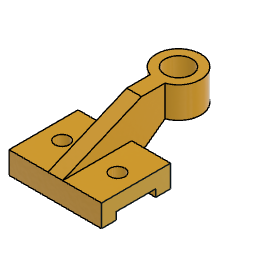
Part (Autodesk Fusion 360 design; units mm, degrees)
Autodesk Fusion 360 part; units mm, degrees
note: some values were not read from the file. Chosen so that the rebuilt part matches the saved one: a side.
sketch "Sketch1" plane through (0, 0, 0) normal (0, 1, 0) x (1, 0, 0)
  line L0 (0, 0) -> (31.5, 0)
  line L1 (31.5, 0) -> (31.5, -18)
  line L2 (31.5, -18) -> (0, -18)
  line L3 (0, -18) -> (0, 0)
  line L4 (0, 0) -> (-6, 0)
  line L5 (-6, 0) -> (-6, -45)
  line L6 (-6, -45) -> (0, -45)
  line L7 (0, -45) -> (0, 0)
  dimension "d1" = 31.5
  dimension "d2" = 18
  dimension "d3" = 6
  dimension "d4" = 45
  constraint horizontal L0
  constraint vertical L1
  constraint horizontal L2
  constraint vertical L3
  constraint coincident L0.start L3.end
  constraint horizontal L4
  constraint vertical L5
  constraint horizontal L6
  constraint vertical L7
  measures "d1" distance of L0.start L0.end
  measures "d2" distance of L0.start L2.end
  measures "d3" distance of L0.start L4.end
  measures "d4" distance of L0.start L6.end
extrude "Extrude1" add sketch "Sketch1" along normal blind 100 contours L3 L4 L5 L6 L7
sketch "Sketch2" plane through (0, 0, 0) normal (0, 1, 0) x (1, 0, 0)
  line L0 (0, 0) -> (31.5, 0)
  line L1 (31.5, 0) -> (31.5, -18)
  line L2 (31.5, -18) -> (0, -18)
  line L3 (0, -18) -> (0, 0)
  dimension "d7" = 31.5
  dimension "d8" = 18
  constraint horizontal L0
  constraint vertical L1
  constraint horizontal L2
  constraint vertical L3
  constraint coincident L0.start L3.end
  measures "d7" distance of L0.start L0.end
  measures "d8" distance of L0.start L2.end
extrude "Extrude2" add sketch "Sketch2" along normal blind 56
sketch "Sketch3" plane through (0, 0, 45) normal (0, 0, 1) x (-1, 0, 0)
  line L0 (6, 0) -> (0, 0)
  line L1 (0, 0) -> (0, -100)
  line L2 (0, -100) -> (6, -100)
  line L3 (6, -100) -> (6, 0)
  arc A0 (6, -82) -> (6, -118) centre (6, -100) ccw
  line L4 (6, -82) -> (6, -118)
  dimension "d11" = 36
  constraint coincident L2.end L3.start
  constraint coincident L3 A0.start
  constraint parallel L3 L4
  measures "d11" diameter of A0
extrude "Extrude3" cut sketch "Sketch3" against normal blind 25 contours L1 L2 L3 A0 L4 | L1 L2 A0 L4
sketch "Sketch4" plane through (0, 0, 45) normal (0, 0, 1) x (-1, 0, 0)
  arc A0 (6, -82) -> (0, -83.0294) centre (6, -100) ccw
  line L0 (6, -82) -> (6, 0)
  line L1 (6, 0) -> (0, 0)
  line L2 (0, 0) -> (0, -83.0294)
  arc A1 (6, -82) -> (6, -118) centre (6, -100) ccw
  dimension "d14" = 36
  constraint concentric A0 A1
  measures "d14" diameter of A1
extrude "Extrude4" add sketch "Sketch4" against normal blind 25 thin wall 7 on the left open curves A1
sketch "Sketch5" plane through (0, 0, 0) normal (1, 0, 0) x (0, 1, 0)
  line L0 (100, 20) -> (90.7805, 20)
  line L1 (90.7805, 20) -> (83.0294, 20)
  line L2 (83.0294, 20) -> (83.0294, 45)
  line L3 (83.0294, 45) -> (0, 45)
  line L4 (0, 45) -> (0, 18)
  line L5 (0, 18) -> (56, 18)
  line L6 (56, 18) -> (56, 0)
  line L7 (56, 0) -> (100, 0)
  line L8 (100, 0) -> (100, 20)
  line L9 (56, 0) -> (83.0294, 20)
  constraint coincident L6.end L7.start
  constraint coincident L1.end L2.start
extrude "Extrude5" cut sketch "Sketch5" against normal blind 15 contours L0 L1 L7 L8 L9
sketch "Sketch6" plane through (0, 0, 0) normal (1, 0, 0) x (0, 1, 0)
  line L0 (56, 0) -> (83.0294, 20)
  line L1 (83.0294, 20) -> (83.0294, 45)
  line L2 (83.0294, 45) -> (0, 45)
  line L3 (0, 45) -> (0, 18)
  line L4 (0, 18) -> (56, 18)
  line L5 (56, 18) -> (56, 0)
  line L6 (0, 45) -> (64, 45)
  line L7 (64, 45) -> (0, 18)
  dimension "d20" = 64
  constraint coincident L2.end L3.start
  constraint perpendicular L3 L6
  constraint coincident L3.end L4.start
  measures "d20" distance of L2.end L6.end
extrude "Extrude6" cut sketch "Sketch6" against normal blind 15 contours L2 L3 L6 L7
sketch "Sketch7" plane through (31.5, 0, 0) normal (1, 0, 0) x (0, 1, 0)
  line L0 (0, 18) -> (0, 0)
  line L1 (0, 0) -> (56, 0)
  line L2 (56, 0) -> (56, 18)
  line L3 (56, 18) -> (0, 18)
  line L4 (12, 0) -> (44, 0)
  line L5 (44, 0) -> (44, 6)
  line L6 (44, 6) -> (12, 6)
  line L7 (12, 6) -> (12, 0)
  dimension "d23" = 12
  dimension "d24" = 32
  dimension "d25" = 6
  constraint horizontal L4
  constraint vertical L5
  constraint horizontal L6
  constraint vertical L7
  measures "d23" distance of L0.end L4.start
  measures "d24" distance of L4.start L4.end
  measures "d25" distance of L4.start L6.end
extrude "Extrude7" cut sketch "Sketch7" against normal blind 65 contours L1 L4 L5 L6 L7
sketch "Sketch8" plane through (31.5, 0, 0) normal (1, 0, 0) x (0, 1, 0)
  line L0 (12, 0) -> (12, 6)
  line L1 (12, 6) -> (44, 6)
  line L2 (44, 6) -> (44, 0)
  line L3 (44, 0) -> (56, 0)
  line L4 (56, 0) -> (56, 18)
  line L5 (56, 18) -> (0, 18)
  line L6 (0, 18) -> (0, 0)
  line L7 (0, 0) -> (12, 0)
hole "Hole1" at (16.5, 28, 18) direction (0, 0, -1) diameter 12 depth 25 tip angle 118
mirror "Mirror1" about plane through (-6, 0, 0) normal (-1, 0, 0) of bodies 1 merged
